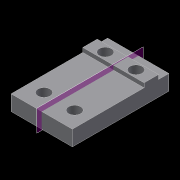
# Autodesk Inventor part: slider manual tension v1
Saved by Autodesk Inventor 2015 SP1 (Build 190203100, 203)
## iProperties
Created: 2014-12-05
Part Number: slider manual tension v1
Material: Generic
Document SubType Name: Modeling
Designer: datenney
Density: 1 g/cm^3
Appearance: Default
Author: datenney
Autodesk Inventor part; units mm, degrees
ref_plane "YZ Plane" through (0, 0, 0) normal (1, 0, 0) x (0, 1, 0)
ref_plane "XZ Plane" through (0, 0, 0) normal (0, 1, 0) x (-1, 0, 0)
ref_plane "XY Plane" through (0, 0, 0) normal (0, 0, 1) x (1, 0, 0)
sketch "Sketch1" plane through (0, 0, 0) normal (0, 1, 0) x (-1, 0, 0)
  line L0 (0, 0) -> (25.4, 0)
  line L1 (25.4, 0) -> (25.4, -40.005)
  line L2 (25.4, -40.005) -> (0, -40.005)
  line L3 (0, -40.005) -> (0, 0)
  dimension "d0" = 40.005
  dimension "d1" = 25.4
  constraints: 8 end point, 2 parallel, 1 horizontal, 1 perpendicular
  measures "d0" distance of L0.end L1.end
  measures "d1" distance between parallel lines of L3 L1
extrude "Extrusion1" add sketch "Sketch1" along normal blind 6.35
sketch "Sketch2" plane through (0, 6.35, 0) normal (0, 1, 0) x (1, 0, 0)
  line L0 (-25.4, 40.005) -> (-25.4, 0) projected
  line L1 (0, 0) -> (0, 40.005) projected
  line L2 (-25.4, 35.6997) -> (0, 35.6997)
  line L3 (0, 35.6997) -> (0, 29.7053)
  line L4 (0, 29.7053) -> (-25.4, 29.7053)
  line L5 (-25.4, 29.7053) -> (-25.4, 35.6997)
  line L6 (-25.4, 32.7025) -> (0, 32.7025) construction
  line L7 (-25.4, 7.3025) -> (0, 7.3025)
  line L8 (-25.4, 0) -> (0, 0) projected
  line L9 (0, 40.005) -> (-25.4, 40.005) projected
  line L10 (-25.4, 29.7053) -> (0, 29.7053)
  line L11 (0, 29.7053) -> (0, 35.6997)
  line L12 (0, 35.6997) -> (-25.4, 35.6997)
  line L13 (-25.4, 35.6997) -> (-25.4, 29.7053)
  line L14 (-12.7, 35.6997) -> (-12.7, 29.7053) construction
  line L15 (-6.35, 7.3025) -> (-6.35, 40.005) construction
  line L16 (-19.05, 7.3025) -> (-19.05, 40.005) construction
  point P0 (-12.7, 32.7025)
  dimension "d4" = 5.9944
  dimension "d5" = 25.4
  dimension "d6" = 7.3025
  dimension "d7" = 40.005
  dimension "d8" = 12.7
  dimension "d9" = 25.4
  dimension "d10" = 6.35
  dimension "d23" = 12.7
  constraints: 26 end point, 8 point on line, 5 midpoint, 4 parallel, 3 horizontal, 2 perpendicular, 2 vertical
  measures "d4" distance between parallel lines of L4 L2
  measures "d5" distance between parallel lines of L6 L7
  measures "d6" distance between parallel lines of L8 L7
  measures "d7" distance between parallel lines of L8 L9
  measures "d8" distance of L16.start L15.start
  measures "d9" distance between parallel lines of L1 L0
  measures "d10" distance of L7.start L16.start
  measures "d23" distance between parallel lines of L3 L14
extrude "Extrusion2" add sketch "Sketch2" along normal blind 5.715 contours L2 L1 L4 L0
hole "Hole1" at (-19.05, 6.35, -7.3025) at (-6.35, 6.35, -7.3025) direction (0, -1, 0) diameter 5 end through all
sketch "Sketch3" plane through (0, 0, 0) normal (1, 0, 0) x (0, 0, -1)
  line L0 (29.7053, 12.065) -> (35.6997, 12.065) projected
  line L1 (40.005, 0) -> (0, 0) projected
  line L2 (40.005, 0) -> (40.005, 6.35) projected
  line L3 (35.6997, 6.35) -> (40.005, 6.35) projected
  line L4 (35.6997, 6.35) -> (35.6997, 12.065) projected
  line L5 (29.7053, 12.065) -> (35.6997, 12.065) projected
  line L6 (29.7053, 6.35) -> (29.7053, 12.065) projected
  line L7 (0, 6.35) -> (29.7053, 6.35) projected
  line L8 (0, 0) -> (0, 6.35) projected
  line L9 (29.7053, 6.35) -> (35.6997, 6.35)
  line L10 (35.6997, 6.35) -> (35.6997, 8.128)
  line L11 (35.6997, 6.35) -> (35.6997, 12.065) projected
  line L12 (35.6997, 8.128) -> (29.7053, 8.128)
  line L13 (29.7053, 8.128) -> (29.7053, 6.35)
  line L14 (29.7053, 8.128) -> (29.7053, 12.065)
  line L15 (29.7053, 12.065) -> (35.6997, 12.065)
  line L16 (35.6997, 12.065) -> (35.6997, 8.128)
  dimension "d20" = 1.778
  constraints: 14 end point, 3 horizontal, 3 vertical, 2 parallel, 2 point on line
  measures "d20" distance between parallel lines of L9 L12
extrude "Extrusion3" cut sketch "Sketch3" against normal through all contours L0 L4 L12 L6
ref_plane "Work Plane1" through (-12.7, 0, -40.005) normal (-1, 0, 0) x (0, 0, 1)
sketch "Sketch4" plane through (0, 8.128, -29.7053) normal (0, 1, 0) x (1, 0, 0)
  circle A0 centre (-6.35, -22.4028) radius 2.5 projected
  circle A1 centre (-19.05, -22.4028) radius 2.5 projected
  line L0 (0, 5.9944) -> (0, 0) projected
  point P0 (0, -29.7053)
  point P1 (-6.35, 2.9972)
  point P2 (-19.05, 2.9972)
  point P3 (0, 2.9972)
  constraints: 2 horizontal alignment, 2 vertical alignment, 1 midpoint
hole "Hole2" at (-6.35, 8.128, -32.7025) at (-19.05, 8.128, -32.7025) direction (0, -1, 0) diameter 5 end through all
equation "\"d6\" = -0.5 * d5 + 0.5 * d7"
equation "\"d10\" = -0.5 * d8 + 0.5 * d9"
equation "\"d24\" = d13"
equation "\"d13\" = 5"
body "Solid1"
